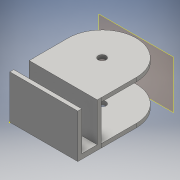
# Autodesk Inventor part: Maintients poullies V4
Saved by Autodesk Inventor 2016 (Build 200138000, 138)
## iProperties
Created: 2016-03-29
Part Number: Maintients poullies V4
Material: Generic
Document SubType Name: Modeling
Designer: Thetheos
Density: 1 g/cm^3
Appearance: Default
Author: Thetheos
Autodesk Inventor part; units mm, degrees
ref_plane "YZ Plane" through (0, 0, 0) normal (1, 0, 0) x (0, 1, 0)
ref_plane "XZ Plane" through (0, 0, 0) normal (0, 1, 0) x (-1, 0, 0)
ref_plane "XY Plane" through (0, 0, 0) normal (0, 0, 1) x (1, 0, 0)
sketch "Sketch1" plane through (0, 0, 0) normal (0, 0, 1) x (1, 0, 0)
  line L0 (0, 0) -> (35, 0)
  line L1 (35, 0) -> (35, 12)
  line L2 (0, 12) -> (0, 0)
  line L3 (0, 12) -> (-0.0372, 12)
  line L4 (35.0398, 12) -> (35, 12)
  line L5 (-0.0372, 12) -> (-0.0372, 30)
  line L6 (35.0398, 12) -> (35.0398, 30)
  arc A0 (35.0398, 30) -> (-0.0372, 30) centre (17.5013, 30) ccw
  circle A1 centre (17.5013, 30) radius 2
  dimension "d0" = 35
  dimension "d1" = 12
  dimension "d4" = 18
  dimension "d6" = 4
  constraints: 14 end point, 2 centre point, 2 point on circle, 2 tangent, 1 coincident, 1 horizontal, 1 perpendicular, 1 vertical
  measures "d0" distance of L0.start L0.end
  measures "d1" distance of L0.end L1.end
  measures "d4" distance of L3.end L5.end
  measures "d6" diameter of A1
extrude "Extrusion1" add sketch "Sketch1" along normal blind 22.5
sketch "Sketch2" plane through (0, 0, 22.5) normal (0, 0, 1) x (1, 0, 0)
  line L0 (0, 2) -> (35, 2)
  line L1 (35, 2) -> (35, 10)
  line L2 (35, 10) -> (0, 10)
  line L3 (0, 10) -> (0, 2)
  point P0 (0, 0)
  constraints: 8 end point, 1 horizontal
extrude "Extrusion2" cut sketch "Sketch2" against normal blind 20
sketch "Sketch3" plane through (-0.0372, 12, 0) normal (-1, 0, 0) x (0, 0, 1)
  point P0 (0, -12)
ref_plane "Work Plane1" through (17.5013, 47.5385, 0) normal (0, -1, 0) x (1, 0, 0)
sketch "Sketch4" plane through (17.5013, 47.5385, 0) normal (0, -1, 0) x (1, 0, 0)
  line L0 (17.5385, 0) -> (17.5385, 22.5) projected
  line L1 (-17.5385, 0) -> (-17.5385, 22.5) projected
  line L2 (17.5385, 20.5) -> (-17.5385, 20.5)
  line L3 (-17.5385, 20.5) -> (-17.5385, 2)
  line L4 (-17.5385, 2) -> (17.5385, 2)
  line L5 (17.5385, 2) -> (17.5385, 20.5)
  line L6 (17.5385, 22.5) -> (-17.5385, 22.5) projected
  point P0 (-17.5013, 0)
  dimension "d11" = 18.5
  dimension "d12" = 2
  constraints: 8 end point, 2 parallel, 2 point on line, 1 horizontal, 1 perpendicular
  measures "d11" distance of L3.end L2.end
  measures "d12" distance between parallel lines of L2 L6
extrude "Extrusion3" cut sketch "Sketch4" along normal blind 35.5 contours L4 L1 L2 L0
body "Solid1"
